Autodesk Fusion 360 part; units mm, degrees
(part 2 of 2)
sketch "Sketch1" plane through (0, 0, 0) normal (0, 0, 1) x (1, 0, 0)
  circle A0 centre (0, 0) radius 11
  circle A1 centre (0, 0) radius 8 construction
  circle A2 centre (0, -8) radius 1.75
  line L0 (0, 0) -> (0, -11) construction
  circle A3 centre (8, 0) radius 1.75
  circle A4 centre (0, 8) radius 1.75
  circle A5 centre (-8, 0) radius 1.75
  circle A6 centre (0, 0) radius 5.1
  circle A7 centre (0, 0) radius 4.05
  dimension "d1" = 22
  dimension "d2" = 16
  dimension "d3" = 3.5
  dimension "d5" = 360
  dimension "d6" = 10.2
  dimension "d7" = 8.1
  constraint coincident A0.centre A1.centre
  constraint coincident A1 A2.centre
  constraint coincident A0 L0.end
  constraint vertical L0
  constraint coincident A2.centre L0
  constraint concentric A0 A7
  measures "d1" diameter of A0
  measures "d2" diameter of A1
  measures "d3" diameter of A2
  measures "d6" diameter of A6
  measures "d7" diameter of A7
extrude "Extrude1" add sketch "Sketch1" along normal blind 3.5 contours A0 | A6 in component "T8 Trapezoidal Nut"
sketch "Sketch2" plane through (0, 0, 3.5) normal (0, 0, 1) x (-1, 0, 0)
  circle A0 centre (0, -8) radius 1.75
  circle A1 centre (8, 0) radius 1.75
  circle A2 centre (0, 8) radius 1.75
  circle A3 centre (-8, 0) radius 1.75
  circle A4 centre (0, 0) radius 11
  circle A5 centre (0, 0) radius 4.05
  circle A6 centre (0, 0) radius 5.1
  circle A7 centre (0, 0) radius 4.05
extrude "Extrude2" add sketch "Sketch2" along normal blind 2 contours A6 in component "T8 Trapezoidal Nut"
extrude "Extrude3" add sketch "Sketch1" against normal blind 9.5 contours A6 in component "T8 Trapezoidal Nut"
fillet "Fillet1" radius 0.5 4 edges at (-10.2556, -3.9778, 0) (-10.2556, -3.9778, 3.5) (-4.7549, 1.8442, -9.5) (4.7549, 1.8442, 5.5) in component "T8 Trapezoidal Nut"
component "T8 Trapezoidal Nut" placed x (1, 0, 0) y (0, 1, 0) z (0, 0, 1) at (0, 0, 0)
equation "d7 = 8 mm + clearance"
equation "clearance = 0.1 mm"

design "FPA_Flange Pillow Block"
Autodesk Fusion 360 part; units mm, degrees
sketch "Sketch1" plane through (0, 0, 0) normal (0, 0, 1) x (1, 0, 0)
  line L0 (0, 0) -> (48, 0) construction
  circle A0 centre (24, 0) radius 13.5
  line L1 (24, 0) -> (42, 0) construction
  circle A1 centre (42, 0) radius 2.5
  line L2 (24, 0) -> (24, -13.5) construction
  circle A2 centre (6, 0) radius 2.5
  line L3 (42, 0) -> (42, -6.4) construction
  line L4 (33.4916, 0) -> (33.4916, -9.6) construction
  line L5 (33.4916, -9.6) -> (42, -6.4)
  line L6 (48, 0) -> (48, -0.682)
  line L7 (44.7601, -5.3619) -> (42, -6.4)
  arc A3 (44.7601, -5.3619) -> (48, -0.682) centre (43, -0.682) ccw
  line L8 (33.4916, 9.6) -> (42, 6.4)
  line L9 (44.7601, 5.3619) -> (42, 6.4)
  arc A4 (48, 0.682) -> (44.7601, 5.3619) centre (43, 0.682) ccw
  line L10 (48, 0) -> (48, 0.682)
  line L11 (14.5084, 9.6) -> (6, 6.4)
  line L12 (3.2399, 5.3619) -> (6, 6.4)
  arc A5 (3.2399, 5.3619) -> (0, 0.682) centre (5, 0.682) ccw
  arc A6 (0, -0.682) -> (3.2399, -5.3619) centre (5, -0.682) ccw
  line L13 (0, 0) -> (0, 0.682)
  line L14 (0, 0) -> (0, -0.682)
  line L15 (3.2399, -5.3619) -> (6, -6.4)
  line L16 (14.5084, -9.6) -> (6, -6.4)
  circle A7 centre (24, 0) radius 4
  circle A8 centre (24, 0) radius 5
  circle A9 centre (24, 0) radius 11.75
  dimension "d1" = 48
  dimension "d2" = 27
  dimension "d3" = 18
  dimension "d4" = 5
  dimension "d5" = 6.4
  dimension "d6" = 9.6
  dimension "d8" = 5
  dimension "d9" = 8
  dimension "d10" = 10
  dimension "d13" = -1.75
  constraint coincident L0.start L13.start
  constraint horizontal L0
  constraint midpoint L0 A0.centre
  constraint coincident A0.centre L1.start
  constraint parallel L0 L1
  constraint coincident L1.end A1.centre
  constraint coincident A0 L2.end
  constraint perpendicular L0 L2
  constraint symmetric A1 L2 A2
  constraint perpendicular L1 L3
  constraint coincident L1 L4.start
  constraint perpendicular L1 L4
  constraint coincident A0 L4.end
  constraint perpendicular L0 L6
  constraint parallel L5 L7
  constraint tangent L7 A3
  constraint tangent L6 A3
  constraint symmetric L0.end L1 L6.start
  constraint symmetric L1 L3.end L8.end
  constraint symmetric L1 L4.end L8.start
  constraint symmetric L1 L7.start L9.start
  constraint symmetric L1 L6.end A4.start
  constraint symmetric L1 A3 A4
  constraint symmetric L0.end L2 L0.start
  constraint symmetric L2 L3.end L15.end
  constraint symmetric L2 L4.end L16.start
  constraint symmetric L2 L7.start A6.end
  constraint symmetric L2 L6.end A6.start
  constraint symmetric L2 A3 A6
  constraint symmetric L2 L8.start L11.start
  constraint symmetric L2 L8.end L11.end
  constraint symmetric L2 L9.start L12.start
  constraint symmetric L2 A4.start A5.end
  constraint symmetric L2 A4 A5
  constraint symmetric L2 L0.end L0.start
  constraint concentric A0 A7
  constraint concentric A7 A8
  measures "d1" distance of L0.start L0.end
  measures "d2" diameter of A0
  measures "d3" distance of A0.centre L1.end
  measures "d4" diameter of A1
  measures "d5" distance of L1.end L3.end
  measures "d6" distance of L4.start L4.end
  measures "d8" radius of A3
  measures "d9" diameter of A7
  measures "d10" diameter of A8
extrude "Extrude1" add sketch "Sketch1" along normal blind 4 contours A0 | A0 L5 L6 L7 A3 L8 L9 A4 L10 | A0 L11 L12 A5 A6 L13 L14 L15 L16 | A8 | A9 in component "Flange Pillow Block"
sketch "Sketch2" plane through (0, 0, 4) normal (0, 0, 1) x (-1, 0, 0)
  circle A0 centre (-24, 0) radius 4
  circle A1 centre (-6, 0) radius 2.5
  circle A2 centre (-42, 0) radius 2.5
  line L0 (-33.4916, 9.6) -> (-44.7601, 5.3619)
  arc A3 (-44.7601, 5.3619) -> (-48, 0.682) centre (-43, 0.682) ccw
  line L1 (-48, 0.682) -> (-48, -0.682)
  arc A4 (-48, -0.682) -> (-44.7601, -5.3619) centre (-43, -0.682) ccw
  line L2 (-44.7601, -5.3619) -> (-33.4916, -9.6)
  arc A5 (-33.4916, -9.6) -> (-14.5084, -9.6) centre (-24, 0) ccw
  line L3 (-14.5084, -9.6) -> (-3.2399, -5.3619)
  arc A6 (-3.2399, -5.3619) -> (0, -0.682) centre (-5, -0.682) ccw
  line L4 (0, -0.682) -> (0, 0.682)
  arc A7 (0, 0.682) -> (-3.2399, 5.3619) centre (-5, 0.682) ccw
  line L5 (-3.2399, 5.3619) -> (-14.5084, 9.6)
  arc A8 (-14.5084, 9.6) -> (-33.4916, 9.6) centre (-24, 0) ccw
  circle A9 centre (-24, 0) radius 13.5
  circle A10 centre (-24, 0) radius 11.75
  circle A11 centre (-24, 0) radius 5
  circle A12 centre (-24, 0) radius 4
extrude "Extrude2" add sketch "Sketch2" along normal blind 4 contours A5 A8 A9 in component "Flange Pillow Block"
extrude "Extrude3" add sketch "Sketch2" along normal blind 8 contours A11 in component "Flange Pillow Block"
extrude "Extrude4" add 1 faces at (14.5624, 0.8322, 4) along direction (0, 0, 1) blind 2 in component "Flange Pillow Block"
component "Flange Pillow Block" placed x (1, 0, 0) y (0, 1, 0) z (0, 0, 1) at (0, 0, 0)
